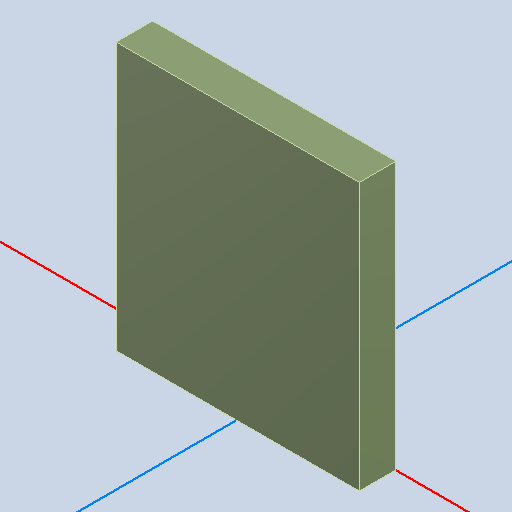
# Autodesk Inventor part: U1_SOT223
Saved by Autodesk Inventor 2022 (Build 260153000, 153)
## iProperties
Created: 2023-03-06
Part Number: U1_SOT223
Material: Типовые
Document SubType Name: Modeling
Designer: Иван Петров
Density: 1 g/cm^3
Appearance: SOT223, U1_SOT223
Author: Иван Петров
Autodesk Inventor part; units mm, degrees
ref_plane "YZ Plane" through (0, 0, 0) normal (1, 0, 0) x (0, 1, 0)
ref_plane "XZ Plane" through (0, 0, 0) normal (0, 1, 0) x (-1, 0, 0)
ref_plane "XY Plane" through (0, 0, 0) normal (0, 0, 1) x (1, 0, 0)
sketch "SOT223, U1_SOT223_12" plane through (0, 0, 0) normal (0, 0, 1) x (1, 0, 0)
  line L0 (-3.2766, 3.6576) -> (3.3782, 3.6576)
  line L1 (3.3782, 3.6576) -> (3.3782, -3.6576)
  line L2 (3.3782, -3.6576) -> (-3.2766, -3.6576)
  line L3 (-3.2766, -3.6576) -> (-3.2766, 3.6576)
  constraints: 8 end point
extrude "Выдавливание1" add sketch "SOT223, U1_SOT223_12" along normal blind 1
